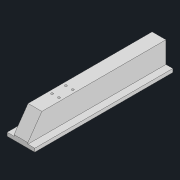
# Autodesk Inventor part: s_base2
Saved by Autodesk Inventor 2021 (Build 250183000, 183)
## iProperties
Created: 2021-08-20
Part Number: s_base2
Material: 一般
Document SubType Name: Modeling
Designer: yuta0
Density: 1 g/cm^3
Appearance: 既定
Author: yuta0
Autodesk Inventor part; units mm, degrees
ref_plane "YZ Plane" through (0, 0, 0) normal (1, 0, 0) x (0, 1, 0)
ref_plane "XZ Plane" through (0, 0, 0) normal (0, 1, 0) x (-1, 0, 0)
ref_plane "XY Plane" through (0, 0, 0) normal (0, 0, 1) x (1, 0, 0)
sketch "スケッチ1" plane through (0, 0, 0) normal (0, 0, 1) x (1, 0, 0)
  line L0 (-20, -2.5) -> (20, -2.5)
  line L1 (20, -2.5) -> (20, 2.5)
  line L2 (-20, 2.5) -> (-20, -2.5)
  line L3 (-20, -2.5) -> (20, 2.5) construction
  line L4 (20, -2.5) -> (-20, 2.5) construction
  line L5 (-10, 2.5) -> (10, 2.5)
  line L6 (10, 2.5) -> (10, 33.5)
  line L7 (10, 33.5) -> (-10, 33.5)
  line L8 (-10, 33.5) -> (-10, 2.5)
  line L9 (-10, 2.5) -> (10, 33.5) construction
  line L10 (10, 2.5) -> (-10, 33.5) construction
  line L11 (20, 2.5) -> (10, 2.5)
  line L12 (-10, 2.5) -> (-20, 2.5)
  point P0 (0, 0)
  point P1 (0, 18)
  point P2 (0, 18)
  point P3 (0, 0)
  dimension "d0" = 20
  dimension "d1" = 31
  dimension "d2" = 5
  dimension "d3" = 10
  constraints: 26 end point, 6 midpoint, 5 parallel, 2 horizontal, 2 perpendicular, 1 vertical alignment
  measures "d0" distance of L6.end L7.end
  measures "d1" distance of L5.end L6.end
  measures "d2" distance of L0.end L1.end
  measures "d3" distance between parallel lines of L8 L2
extrude "押し出し1" add sketch "スケッチ1" along normal mid plane 200
sketch "スケッチ4" plane through (20, -2.5, 100) normal (1, 0, 0) x (0, 0, -1)
  line L0 (0, 7) -> (20.306, 36)
  line L1 (200, 36) -> (0, 36) projected
  line L2 (0, 5) -> (0, 36) projected
  line L3 (200, 5) -> (0, 5) projected
  line L4 (200, 36) -> (200, 5) projected
  line L5 (0, 0) -> (0, 5) projected
  point P0 (100, 2.5)
  dimension "d18" = 35
  dimension "d21" = 2
  constraints: 2 end point, 2 point on line
  measures "d18" angle of L2 L0
  measures "d21" distance from line of L3 L0.start
extrude "押し出し3" cut sketch "スケッチ4" against normal through all contours L2 L1 L0
sketch "スケッチ5" plane through (-10, -2.5, -100) normal (0, 1, 0) x (1, 0, 0)
  line L0 (20, -200) -> (0, -200) projected
  line L1 (0, 0) -> (0, -179.694) projected
  line L2 (20, 0) -> (20, -179.694) projected
  point P0 (10, -100)
  point P1 (5, -150)
  point P2 (5, -130)
  point P3 (15, -130)
  point P4 (15, -150)
  dimension "d22" = 50
  dimension "d23" = 20
  dimension "d24" = 5
  dimension "d25" = 5
  constraints: 2 horizontal alignment, 2 vertical alignment
  measures "d22" distance from line of L0 point (5, -150)
  measures "d23" distance of point (5, -130) point (5, -150)
  measures "d24" distance from line of L1 point (5, -150)
  measures "d25" distance from line of L2 point (15, -130)
hole "穴2" at (-5, -2.5, 50) at (-5, -2.5, 30) at (5, -2.5, 30) at (5, -2.5, 50) direction (0, 1, 0) diameter 3.2 end through all counterbore diameter 6.5 counterbore depth 3 clearance for "Socket Head Cap Screw" size "M3" standard "Ansi Metric M Profile"
